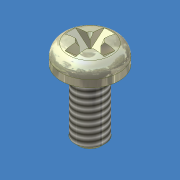
# Autodesk Inventor part: Phillips Pan Head Machine Screw Inch
Saved by Autodesk Inventor 2013 (Build 170138000, 138)
## iProperties
Shininess: 70.0
Length Units: 11272
Angle Units: 11279
Time Units: 11290
Mass Units: 11286
Length Display Precision: 3
Angle Display Precision: 2
Created: 2000-12-30
Part Number: Phillips Pan Head Machine Screw Inch
Document SubType Name: Modeling
Designer: Administrator
Material: Steel, High Strength Low Alloy
Density: 7.84 g/cm^3
Density: 7.84
Volumn: 0.0334175022831377
Area: 0.7931629180511741
PropertySet Name: Model Information
Control State: 0
Master: False
Checked Out: False
HeadHeight: 0.110 in
Author: Administrator
Autodesk Inventor part; units mm, degrees
ref_plane "YZ Plane" through (0, 0, 0) normal (1, 0, 0) x (0, 1, 0)
ref_plane "XZ Plane" through (0, 0, 0) normal (0, 1, 0) x (-1, 0, 0)
ref_plane "XY Plane" through (0, 0, 0) normal (0, 0, 1) x (1, 0, 0)
sketch "Sketch1" plane through (0, 0, 0) normal (0, 0, 1) x (1, 0, 0)
  line L0 (0, -5.4574) -> (0, 4.0933) projected
  line L1 (2.1209, 0) -> (2.1209, 0.5237)
  arc A0 (2.1209, 0.5237) -> (1.5692, 1.3462) centre (1.2319, 0.5237) ccw
  arc A1 (1.5692, 1.3462) -> (0.7645, 1.5048) centre (0.7645, -0.6161) ccw
  line L2 (0.7645, 1.5048) -> (0, 1.5048)
  line L3 (2.1209, 0) -> (1.0922, 0)
  line L4 (1.0922, 0) -> (1.0922, -4.7752)
  line L5 (1.0922, -4.7752) -> (0, -4.7752)
  point P0 (0, 0)
  dimension "d0" = 2.1844
  dimension "d1" = 4.2418
  dimension "d2" = 0.889
  dimension "d3" = 2.1209
  dimension "d4" = 4.7752
  dimension "d6" = 1.5291
  dimension "d8" = 1.3462
  constraints: 10 end point, 4 point on circle, 3 perpendicular, 3 point on line, 3 tangent, 2 centre point, 2 parallel
  measures "d0" diameter of L4 L0
  measures "d1" diameter of L1 L0
  measures "d2" radius of A0
  measures "d3" radius of A1
  measures "d4" distance of L3.end L4.end
  measures "d6" diameter of L2.start L0
  measures "d8" distance from line of L3 A0.end
revolve "Revolution1" add sketch "Sketch1" angle 360 about axis through (0, -10, 0) along (0, 1, 0)
sketch "Sketch2" plane through (0, 0, 0) normal (0, 0, 1) x (1, 0, 0)
  line L0 (0, 0.1586) -> (-1.5907, 1.5048)
  line L1 (-1.5907, 1.5048) -> (1.5907, 1.5048)
  line L2 (1.5907, 1.5048) -> (0, 0.1586)
  line L3 (0, 0.0835) -> (0, 2.5016) projected
  line L4 (-0.7645, 1.5048) -> (0.7645, 1.5048) projected
  dimension "d9" = 3.1814
  dimension "d22" = 1.3462
  constraints: 6 end point, 1 collinear, 1 equal length, 1 horizontal, 1 point on line
  measures "d9" distance of L0.end L1.end
  measures "d22" distance from line of L1 L0.start
extrude "Extrusion1" cut sketch "Sketch2" against normal mid plane 0.7874
sketch "Sketch3" plane through (0, 0, 0) normal (1, 0, 0) x (0, 1, 0)
  line L0 (1.5048, 1.5907) -> (1.5048, -1.5907)
  line L1 (1.5048, -1.5907) -> (0.1586, 0)
  line L2 (0.1586, 0) -> (1.5048, 1.5907)
  point P0 (1.5048, 0)
  point P1 (1.5048, 0)
  point P2 (1.5048, 0)
  dimension "d12" = 3.1814
  constraints: 6 end point, 1 equal length, 1 midpoint, 1 vertical
  measures "d12" distance of L0.start L0.end
extrude "Extrusion2" cut sketch "Sketch3" against normal mid plane 0.7874
sketch "Sketch4" plane through (-0.6554, 1.5048, 0.3937) normal (0, 1, 0) x (1, 0, 0)
  arc A0 (0, 0) -> (0.2617, -0.2617) centre (0.6554, 0.3937) ccw projected
  circle A1 centre (0.6554, 0.3937) radius 0.7645
  dimension "d17" = 1.5291
  constraints: 1 coincident, 2 other
extrude "Extrusion3" cut sketch "Sketch4" against normal blind 0.7645 draft -30
thread "Thread1" size "2-56 UNC" class "2A" standard "ANSI Unified Screw Threads" length 4.5466
chamfer "Chamfer1" distance 0.2731 angle 45 1 edges at (-1.0922, -4.7752, 0)
equation "\"d0\" = Dia"
equation "\"d1\" = HeadDia"
equation "\"d2\" = HeadRad"
equation "\"d3\" = 0.5 * d1"
equation "\"d4\" = ShankLength"
equation "\"d6\" = 0.7 * d0"
equation "\"d8\" = HeadHeight"
equation "\"d9\" = 0.75 * d1"
equation "\"d22\" = HeadHeight"
equation "\"d10\" = SlotW"
equation "\"d12\" = d9"
equation "\"d13\" = SlotW"
equation "\"d17\" = d6"
equation "\"d15\" = 0.5 * d6"
equation "\"d18\" = ThreadLength"
equation "\"d20\" = 0.125 * Dia"
equation "\"d21\" = 0.125 * Dia"
equation "\"Dia\" = 2.1844"
equation "\"ShankLength\" = 4.7752"
equation "\"HeadDia\" = 4.2418"
equation "\"HeadRad\" = 0.889"
equation "\"SlotW\" = 0.7874"
equation "\"SlotD\" = 0.7874"
equation "\"HeadHeight\" = 1.3462"
equation "\"ThreadLength\" = 4.5466"
body "Solid1"
